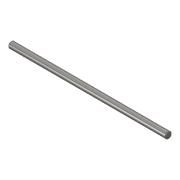
# Autodesk Inventor part: SUS-Shaft
Saved by Autodesk Inventor 2019.4 (Build 234330000, 330)
## iProperties
Created: 2020-02-15
Part Number: SUS-Shaft
Material: Steel, Alloy
Document SubType Name: Modeling
Designer: Lord of Xy
Density: 7.73 g/cm^3
Appearance: Semi-Polished
Mass: 310.187 g
Surface Area: 128.403 cm^2
Volume: 40.1277 cm^3
Author: Lord of Xy
Autodesk Inventor part; units mm, degrees
ref_plane "YZ Plane" through (0, 0, 0) normal (1, 0, 0) x (0, 1, 0)
ref_plane "XZ Plane" through (0, 0, 0) normal (0, 1, 0) x (-1, 0, 0)
ref_plane "XY Plane" through (0, 0, 0) normal (0, 0, 1) x (1, 0, 0)
sketch "Sketch1" plane through (0, 0, 0) normal (1, 0, 0) x (0, 1, 0)
  circle A0 centre (0, 0) radius 6.35
  dimension "d0" = 12.7
  constraints: 1 centre point, 1 coincident
  measures "d0" diameter of A0
extrude "Extrusion1" add sketch "Sketch1" along normal mid plane 317.5
chamfer "Chamfer1" distance 1.5875 angle 45 2 edges at (158.75, -6.35, 0) (-158.75, -6.35, 0)
body "Solid1"
